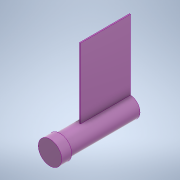
# Autodesk Inventor part: portionOfShade
Saved by Autodesk Inventor 2021.2 (Build 252289000, 289)
## iProperties
Created: 2021-02-12
Part Number: portionOfShade
Material: PC/ABS Plastic
Document SubType Name: Modeling
Designer: robst
Density: 0.357273 g/cm^3
Appearance: Smooth - Purple
Author: robst
Autodesk Inventor part; units mm, degrees
ref_plane "YZ Plane" through (0, 0, 0) normal (1, 0, 0) x (0, 1, 0)
ref_plane "XZ Plane" through (0, 0, 0) normal (0, 1, 0) x (-1, 0, 0)
ref_plane "XY Plane" through (0, 0, 0) normal (0, 0, 1) x (1, 0, 0)
sketch "Sketch1" plane through (0, 0, 0) normal (0, 0, 1) x (1, 0, 0)
  circle A0 centre (0, 0) radius 6.35
  dimension "d0" = 12.7
  constraints: 1 centre point, 1 coincident
  measures "d0" diameter of A0
extrude "Extrusion1" add sketch "Sketch1" against normal blind 50.8
sketch "Sketch2" plane through (0, 0, 0) normal (0, 0, 1) x (1, 0, 0)
  circle A0 centre (0, 0) radius 7.4295
  dimension "d3" = 14.859
  constraints: 1 centre point, 1 coincident
  measures "d3" diameter of A0
extrude "Extrusion3" add sketch "Sketch2" against normal blind 6.35
sketch "Sketch3" plane through (0, 0, 0) normal (1, 0, 0) x (0, 1, 0)
  line L0 (-6.35, -50.8) -> (6.35, -50.8) projected
  line L1 (0, -50.8) -> (50.8, -50.8)
  line L2 (50.8, -50.8) -> (50.8, -19.05)
  line L3 (50.8, -19.05) -> (0, -19.05)
  line L4 (0, -19.05) -> (0, -50.8)
  line L5 (7.4295, 0) -> (-7.4295, 0) projected
  point P0 (0, 0)
  dimension "d8" = 19.05
  dimension "d9" = 50.8
  constraints: 8 end point, 2 parallel, 1 horizontal, 1 midpoint, 1 perpendicular
  measures "d8" distance between parallel lines of L3 L5
  measures "d9" distance of L1.start L1.end
extrude "Extrusion4" add sketch "Sketch3" along normal mid plane 0.635
body "Solid1"
